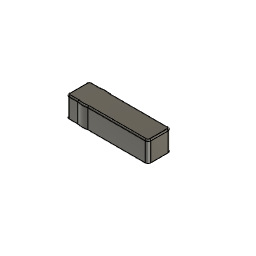
遮光罩 (Autodesk Fusion 360 design; units mm, degrees)
Autodesk Fusion 360 part; units mm, degrees
sketch "草图1" plane through (0, 0, 6) normal (0, 0, 1) x (-1, 0, 0)
  line L0 (-74.3556, -25.6937) -> (-99.7556, -25.6937)
  line L1 (-99.7556, -25.6937) -> (-99.7556, -0.2937)
  line L2 (-99.7556, -0.2937) -> (-74.3556, -0.2937)
  line L3 (-74.3556, -0.2937) -> (-74.3556, -25.6937)
  line L4 (-98, -27.5) -> (-2, -27.5)
  arc A0 (-2, -27.5) -> (1.5, -24) centre (-2, -24) ccw
  line L5 (1.5, -24) -> (1.5, -2)
  arc A1 (1.5, -2) -> (-2, 1.5) centre (-2, -2) ccw
  line L6 (-2, 1.5) -> (-98, 1.5)
  arc A2 (-98, 1.5) -> (-101.5, -2) centre (-98, -2) ccw
  line L7 (-101.5, -2) -> (-101.5, -24)
  arc A3 (-101.5, -24) -> (-98, -27.5) centre (-98, -24) ccw
  line L8 (-2, 0) -> (-98, 0)
  arc A4 (-98, 0) -> (-100, -2) centre (-98, -2) ccw
  line L9 (-100, -2) -> (-100, -24)
  arc A5 (-100, -24) -> (-98, -26) centre (-98, -24) ccw
  line L10 (-98, -26) -> (-2, -26)
  arc A6 (-2, -26) -> (0, -24) centre (-2, -24) ccw
  line L11 (0, -24) -> (0, -2)
  arc A7 (0, -2) -> (-2, 0) centre (-2, -2) ccw
  dimension "d130" = -1.5
extrude "拉伸1" add sketch "草图1" along normal blind 24
sketch "草图2" plane through (0, 0, 30) normal (0, 0, 1) x (-1, 0, 0)
  arc A0 (-101.5, -24) -> (-98, -27.5) centre (-98, -24) ccw
  line L0 (-98, -27.5) -> (-2, -27.5)
  arc A1 (-2, -27.5) -> (1.5, -24) centre (-2, -24) ccw
  line L1 (1.5, -24) -> (1.5, -2)
  arc A2 (1.5, -2) -> (-2, 1.5) centre (-2, -2) ccw
  line L2 (-2, 1.5) -> (-98, 1.5)
  arc A3 (-98, 1.5) -> (-101.5, -2) centre (-98, -2) ccw
  line L3 (-101.5, -2) -> (-101.5, -24)
extrude "拉伸2" add sketch "草图2" along normal blind 1.5
sketch "草图3" plane through (0, 0, 6) normal (0, 0, 1) x (-1, 0, 0)
  arc A0 (-25.6091, -27.5) -> (-12.9225, -27.5) centre (-19.2658, -1.7704) ccw
  line L0 (-12.9225, -27.5) -> (-2, -27.5)
  arc A1 (-2, -27.5) -> (1.5, -24) centre (-2, -24) ccw
  line L1 (1.5, -24) -> (1.5, -2)
  arc A2 (1.5, -2) -> (-2, 1.5) centre (-2, -2) ccw
  line L2 (-2, 1.5) -> (-12.9225, 1.5)
  arc A3 (-12.9225, 1.5) -> (-25.6091, 1.5) centre (-19.2658, -25.2584) ccw
  line L3 (-25.6091, 1.5) -> (-98, 1.5)
  arc A4 (-98, 1.5) -> (-101.5, -2) centre (-98, -2) ccw
  line L4 (-101.5, -2) -> (-101.5, -24)
  arc A5 (-101.5, -24) -> (-98, -27.5) centre (-98, -24) ccw
  line L5 (-98, -27.5) -> (-73.2, -27.5)
  line L6 (-73.2, -27.5) -> (-25.6091, -27.5)
  line L7 (-17.6545, -27.5) -> (-20.8771, -27.5)
  line L8 (-20.8771, -27.5) -> (-20.8771, 1.5)
  line L9 (-20.8771, 1.5) -> (-17.6545, 1.5)
  line L10 (-17.6545, 1.5) -> (-17.6545, -27.5)
  line L11 (-74.3556, -25.6937) -> (-99.7556, -25.6937)
  line L12 (-99.7556, -25.6937) -> (-99.7556, -0.2937)
  line L13 (-99.7556, -0.2937) -> (-74.3556, -0.2937)
  line L14 (-74.3556, -0.2937) -> (-74.3556, -25.6937)
  line L15 (-12.9225, 1.5) -> (-25.6091, 1.5)
  line L16 (-12.9225, -27.5) -> (-25.6091, -27.5)
  arc A6 (-25.6091, -27.5) -> (-12.9225, -27.5) centre (-19.2658, -1.7704) ccw
  arc A7 (-12.9225, 1.5) -> (-25.6091, 1.5) centre (-19.2658, -25.2584) ccw
  constraint coincident L2.end A3.start
  constraint coincident A3.end L3.start
  constraint coincident A0.end L0.start
  constraint coincident A0.start L6.end
extrude "拉伸3" add sketch "草图3" along normal up to surface (25.5 mm away) contours A0 L7 L16 A6 | A3 L9 L15 A7
fillet "圆角1" radius 1.5 12 edges at (61.8046, -1.5, 31.5) (100.4749, -0.4749, 31.5) (101.5, 13, 31.5) (100.4749, 26.4749, 31.5) (61.8046, 27.5, 31.5) (19.2658, -2.2416, 31.5) (7.4612, 27.5, 31.5) (-0.4749, 26.4749, 31.5) (-1.5, 13, 31.5) (-0.4749, -0.4749, 31.5) (7.4612, -1.5, 31.5) (19.2658, 28.2704, 31.5)
